Autodesk Fusion 360 part; units mm, degrees
(part 5 of 5)
sketch "Skizze81" plane through (0, 10, 0) normal (0, -1, 0) x (1, 0, 0)
  line L0 (-37.5877, 27.75) -> (-34.4123, 27.75)
  line L1 (-34.4123, 27.75) -> (-32.8246, 25)
  line L2 (-32.8246, 25) -> (-34.4123, 22.25)
  line L3 (-34.4123, 22.25) -> (-37.5877, 22.25)
  line L4 (-37.5877, 22.25) -> (-39.1754, 25)
  line L5 (-39.1754, 25) -> (-37.5877, 27.75)
  line L6 (-32.5, 27.5) -> (-33.8276, 28.3587)
  arc A0 (-33.8276, 28.3587) -> (-36.0513, 21.0003) centre (-36, 25) ccw
  arc A1 (-34.4939, 20.8944) -> (-36.0513, 21.0003) centre (-36.233, 6.8289) ccw
  line L7 (-34.4939, 20.8944) -> (-34.4939, 21.2944)
  arc A2 (-34.4939, 21.2944) -> (-32.6769, 27.2265) centre (-36, 25) ccw
  line L8 (-32.6769, 27.2265) -> (-32.5, 27.5)
  circle A3 centre (-36, 25) radius 4
  line L9 (-34.4123, -27.75) -> (-37.5877, -27.75)
  line L10 (-37.5877, -27.75) -> (-39.1754, -25)
  line L11 (-39.1754, -25) -> (-37.5877, -22.25)
  line L12 (-37.5877, -22.25) -> (-34.4123, -22.25)
  line L13 (-34.4123, -22.25) -> (-32.8246, -25)
  line L14 (-32.8246, -25) -> (-34.4123, -27.75)
  arc A4 (-36.0513, -21.0003) -> (-33.8276, -28.3587) centre (-36, -25) ccw
  line L15 (-33.8276, -28.3587) -> (-32.5, -27.5)
  line L16 (-32.5, -27.5) -> (-32.6769, -27.2265)
  arc A5 (-32.6769, -27.2265) -> (-34.4939, -21.2944) centre (-36, -25) ccw
  line L17 (-34.4939, -21.2944) -> (-34.4939, -20.8944)
  arc A6 (-36.0513, -21.0003) -> (-34.4939, -20.8944) centre (-36.233, -6.8289) ccw
  circle A7 centre (-36, 25) radius 1.9
  arc A8 (-33.8276, 28.3587) -> (-36.0513, 21.0003) centre (-36, 25) ccw
  line L18 (-33.8276, 28.3587) -> (-32.5, 27.5)
  line L19 (-32.5, 27.5) -> (32.5, 27.5)
  line L20 (32.5, 27.5) -> (32.5, 19)
  line L21 (32.5, 19) -> (31, 19)
  line L22 (31, 19) -> (31, 26)
  line L23 (31, 26) -> (-31, 26)
  line L24 (-31, 26) -> (-31, 20)
  arc A9 (-31, 20) -> (-36.0513, 21.0003) centre (-36.233, 6.8289) ccw
  circle A10 centre (-36, 25) radius 1.9
  line L25 (-45.682, 18.318) -> (-44.6213, 17.2574)
  line L26 (-44.6213, 17.2574) -> (-41.8787, 20)
  line L27 (-41.8787, 20) -> (-31, 20)
  line L28 (-31, 20) -> (-31, 26)
  line L29 (-31, 26) -> (31, 26)
  line L30 (31, 26) -> (31, 19.2)
  line L31 (31, 19.2) -> (32.5, 19.2)
  line L32 (32.5, 19.2) -> (32.5, 27.5)
  line L33 (32.5, 27.5) -> (-32.5, 27.5)
  line L34 (-32.5, 27.5) -> (-33.8276, 28.3587)
  arc A11 (-33.8276, 28.3587) -> (-39.5022, 26.9326) centre (-36, 25) ccw
  line L35 (-39.5022, 26.9326) -> (-42.5, 21.5)
  line L36 (-42.5, 21.5) -> (-45.682, 18.318)
  circle A12 centre (-36, 25) radius 1.9
  line L37 (-47.8033, 16.1967) -> (-45.682, 18.318)
  line L38 (-47.8033, 16.1967) -> (-46.7426, 15.136)
  line L39 (-44.6213, 17.2574) -> (-46.7426, 15.136)
  line L40 (-44.6213, 17.2574) -> (-45.682, 18.318)
  line L41 (-57.5, 6.5) -> (-47.8033, 16.1967)
  line L42 (-46.7426, 15.136) -> (-47.8033, 16.1967)
  line L43 (-47.8033, 16.1967) -> (-57.5, 6.5)
  line L44 (-57.5, 6.5) -> (-57.5, 4)
  line L45 (-57.5, 4) -> (-51.5218, 4)
  line L46 (-51.5218, 4) -> (-51.5218, 10.3569)
  line L47 (-51.5218, 10.3569) -> (-46.7426, 15.136)
  line L48 (-51.5218, 4) -> (-57.5, 4)
  line L49 (-57.5, -4) -> (-57.5, 4)
  line L50 (-57.5, -4) -> (-51.5218, -4)
  line L51 (-51.5218, 4) -> (-51.5218, -4)
  line L52 (-47.8033, -16.1967) -> (-46.7426, -15.136)
  line L53 (-46.7426, -15.136) -> (-51.5218, -10.3569)
  line L54 (-51.5218, -10.3569) -> (-51.5218, -4)
  line L55 (-51.5218, -4) -> (-57.5, -4)
  line L56 (-57.5, -4) -> (-57.5, -6.5)
  line L57 (-57.5, -6.5) -> (-47.8033, -16.1967)
  line L58 (-45.682, -18.318) -> (-47.8033, -16.1967)
  line L59 (-45.682, -18.318) -> (-44.6213, -17.2574)
  line L60 (-46.7426, -15.136) -> (-44.6213, -17.2574)
  line L61 (-46.7426, -15.136) -> (-47.8033, -16.1967)
  circle A13 centre (-36, -25) radius 1.9
  line L62 (-44.6213, -17.2574) -> (-45.682, -18.318)
  line L63 (-45.682, -18.318) -> (-42.5, -21.5)
  line L64 (-42.5, -21.5) -> (-39.5022, -26.9326)
  arc A14 (-39.5022, -26.9326) -> (-33.8276, -28.3587) centre (-36, -25) ccw
  line L65 (-33.8276, -28.3587) -> (-32.5, -27.5)
  line L66 (-32.5, -27.5) -> (-18.7617, -27.5)
  line L67 (-18.7617, -27.5) -> (-18.7617, -26)
  line L68 (-18.7617, -26) -> (-23, -26)
  line L69 (-23, -26) -> (-31, -26)
  line L70 (-31, -26) -> (-31, -20)
  line L71 (-31, -20) -> (-41.8787, -20)
  line L72 (-41.8787, -20) -> (-44.6213, -17.2574)
  circle A15 centre (-36, -25) radius 4
  arc A16 (-36.0513, 21.0003) -> (-41.8787, 20) centre (-36.2598, 4.7412) ccw
  arc A17 (-41.8787, -20) -> (-36.0513, -21.0003) centre (-36.2598, -4.7412) ccw
  constraint concentric A0 A3
  constraint concentric A4 A15
  constraint tangent A4 A15
  constraint tangent A0 A3
  constraint coincident A0.end A1.end
  constraint coincident L26.end L27.start
  constraint tangent A3 A16
  constraint coincident A4.start A6.start
  constraint coincident L71.end L72.start
  constraint tangent A15 A17
extrude "Extrusion94" add sketch "Skizze81" along normal blind 10 separate body contours L0 L1 L2 L3 L4 L5 | A0 A2 A3 A8 A11 | A0 A3 A8 L25 L26 L35 L36 L40 A16 | L25 L37 L38 L39 L40 L42 | L38 L41 L42 L43 L44 L45 L46 L47 L48 | L45 L48 L49 L50 L51 L55 | L50 L52 L53 L54 L55 L56 L57 L61 | L52 L58 L59 L60 L61 L62 | A4 L59 L62 L63 L64 L72 A15 A17 | A4 A5 A14 A15 | L9 L10 L11 L12 L13 L14 makes body 4
sketch "Skizze82" plane through (0, 10, 0) normal (0, 1, 0) x (-1, 0, 0)
  circle A0 centre (36, -25) radius 1.9
  circle A1 centre (36, 25) radius 1.9
  line L0 (51.5218, -10.3569) -> (41.8787, -20)
  arc A2 (36.0513, -21.0003) -> (41.8787, -20) centre (36.2598, -4.7412) ccw
  arc A3 (36.0513, -21.0003) -> (39.5022, -26.9326) centre (36, -25) ccw
  line L1 (39.5022, -26.9326) -> (42.5, -21.5)
  line L2 (42.5, -21.5) -> (57.5, -6.5)
  line L3 (57.5, -6.5) -> (57.5, 6.5)
  line L4 (57.5, 6.5) -> (42.5, 21.5)
  line L5 (42.5, 21.5) -> (39.5022, 26.9326)
  arc A4 (39.5022, 26.9326) -> (36.0513, 21.0003) centre (36, 25) ccw
  arc A5 (41.8787, 20) -> (36.0513, 21.0003) centre (36.2598, 4.7412) ccw
  line L6 (41.8787, 20) -> (51.5218, 10.3569)
  line L7 (51.5218, 10.3569) -> (51.5218, -10.3569)
  arc A6 (36.0513, 21.0003) -> (33.8276, 28.3587) centre (36, 25) ccw
  line L8 (33.8276, 28.3587) -> (32.5, 27.5)
  line L9 (32.5, 27.5) -> (-32.5, 27.5)
  line L10 (-32.5, 27.5) -> (-32.5, 19)
  line L11 (-32.5, 19) -> (-31, 19)
  line L12 (-31, 19) -> (-31, 26)
  line L13 (-31, 26) -> (31, 26)
  line L14 (31, 26) -> (31, 20)
  arc A7 (36.0513, 21.0003) -> (31, 20) centre (36.233, 6.8289) ccw
  circle A8 centre (36, 25) radius 1.9
  circle A9 centre (36, -25) radius 1.9
  circle A10 centre (36, 25) radius 1.9
  line L15 (41.8787, -20) -> (51.5218, -10.3569)
  line L16 (51.5218, -10.3569) -> (51.5218, 10.3569)
  line L17 (51.5218, 10.3569) -> (41.8787, 20)
  arc A11 (41.8787, 20) -> (36.0513, 21.0003) centre (36.2598, 4.7412) ccw
  arc A12 (39.5022, 26.9326) -> (36.0513, 21.0003) centre (36, 25) ccw
  line L18 (39.5022, 26.9326) -> (42.5, 21.5)
  line L19 (42.5, 21.5) -> (57.5, 6.5)
  line L20 (57.5, 6.5) -> (57.5, -6.5)
  line L21 (57.5, -6.5) -> (42.5, -21.5)
  line L22 (42.5, -21.5) -> (39.5022, -26.9326)
  arc A13 (36.0513, -21.0003) -> (39.5022, -26.9326) centre (36, -25) ccw
  arc A14 (36.0513, -21.0003) -> (41.8787, -20) centre (36.2598, -4.7412) ccw
  circle A15 centre (36, -25) radius 1.9
  arc A16 (33.8276, -28.3587) -> (36.0513, -21.0003) centre (36, -25) ccw
  arc A17 (31, -20) -> (36.0513, -21.0003) centre (36.233, -6.8289) ccw
  line L23 (31, -20) -> (31, -26)
  line L24 (31, -26) -> (18.7617, -26)
  line L25 (18.7617, -26) -> (18.7617, -27.5)
  line L26 (18.7617, -27.5) -> (32.5, -27.5)
  line L27 (32.5, -27.5) -> (33.8276, -28.3587)
  line L28 (39.9936, -25.2256) -> (40.3068, -25.4745)
  line L29 (37.6237, -21.3444) -> (37.6237, -20.9444)
  line L30 (0, 1.75) -> (0, 22.5)
  line L31 (-1.75, 0) -> (-22.5, 0)
  line L32 (39.9936, 25.2256) -> (40.3068, 25.4745)
  line L33 (37.6237, 21.3444) -> (37.6237, 20.9444)
  dimension "d393" = 0.4
  dimension "d394" = 0.4
  constraint coincident A16 L28.start
  constraint coincident L22 L28.end
  constraint coincident A16 L29.start
  constraint coincident A14 L29.end
  constraint parallel L29 L30
  constraint symmetric L28.start L31 L32.start
  constraint symmetric L28.end L31 L32.end
  constraint symmetric L29.start L31 L33.start
  constraint symmetric L29.end L31 L33.end
  measures "d393" distance of L28.start L28.end
  measures "d394" vertical distance of L29.start L29.end
extrude "Extrusion95" add sketch "Skizze82" along normal blind 9 contours L0 A2 L1 L2 L3 L4 L5 A5 L6 L7 A6 L15 L16 L17 A11 L18 L19 L20 L21 L22 A14 A16 L28 L29 L32 L33 bodies 4
sketch "Skizze83" plane through (0, 0, 0) normal (0, -1, 0) x (1, 0, 0)
  circle A0 centre (-36, -25) radius 1.9
  circle A1 centre (-36, 25) radius 1.9
  line L0 (-41.8787, -20) -> (-51.5218, -10.3569)
  line L1 (-51.5218, -10.3569) -> (-51.5218, 10.3569)
  line L2 (-51.5218, 10.3569) -> (-41.8787, 20)
  arc A2 (-36.0513, 21.0003) -> (-41.8787, 20) centre (-36.2598, 4.7412) ccw
  arc A3 (-36.0513, 21.0003) -> (-39.5022, 26.9326) centre (-36, 25) ccw
  line L3 (-39.5022, 26.9326) -> (-42.5, 21.5)
  line L4 (-42.5, 21.5) -> (-57.5, 6.5)
  line L5 (-57.5, 6.5) -> (-57.5, -6.5)
  line L6 (-57.5, -6.5) -> (-42.5, -21.5)
  line L7 (-42.5, -21.5) -> (-39.5022, -26.9326)
  arc A4 (-39.5022, -26.9326) -> (-36.0513, -21.0003) centre (-36, -25) ccw
  arc A5 (-41.8787, -20) -> (-36.0513, -21.0003) centre (-36.2598, -4.7412) ccw
  arc A6 (-31, -20) -> (-31, 20) centre (-45.151, 0) ccw
  arc A7 (-31, 20) -> (-34.4939, 20.8944) centre (-36.233, 6.8289) ccw
  arc A8 (-34.4939, -20.8944) -> (-31, -20) centre (-36.233, -6.8289) ccw
  arc A9 (-36.0513, -21.0003) -> (-34.4939, -20.8944) centre (-36.233, -6.8289) ccw
  arc A10 (-36.0513, 21.0003) -> (-39.5022, 26.9326) centre (-36, 25) ccw
  arc A11 (-34.4939, 20.8944) -> (-36.0513, 21.0003) centre (-36.233, 6.8289) ccw
  arc A12 (-39.9936, 25.2256) -> (-37.6237, 21.3444) centre (-36, 25) ccw
  line L8 (-37.6237, 21.3444) -> (-37.6237, 20.9444)
  arc A13 (-37.6237, 20.9444) -> (-41.8787, 20) centre (-36.2598, 4.7412) ccw
  line L9 (-41.8787, 20) -> (-51.5218, 10.3569)
  line L10 (-51.5218, 10.3569) -> (-51.5218, -10.3569)
  line L11 (-51.5218, -10.3569) -> (-41.8787, -20)
  arc A14 (-41.8787, -20) -> (-37.6237, -20.9444) centre (-36.2598, -4.7412) ccw
  line L12 (-37.6237, -20.9444) -> (-37.6237, -21.3444)
  arc A15 (-37.6237, -21.3444) -> (-39.9936, -25.2256) centre (-36, -25) ccw
  line L13 (-39.9936, -25.2256) -> (-40.3068, -25.4745)
  line L14 (-40.3068, -25.4745) -> (-42.5, -21.5)
  line L15 (-42.5, -21.5) -> (-57.5, -6.5)
  line L16 (-57.5, -6.5) -> (-57.5, 6.5)
  line L17 (-57.5, 6.5) -> (-42.5, 21.5)
  line L18 (-42.5, 21.5) -> (-40.3068, 25.4745)
  line L19 (-40.3068, 25.4745) -> (-39.9936, 25.2256)
extrude "Extrusion96" add sketch "Skizze83" against normal blind 3 contours L0 L1 L2 A2 A5 A6 A7 A8 A9 A11 A13 L9 L10 L11 A14 bodies 4
sketch "Skizze84" plane through (-57.5, 0, 0) normal (-1, 0, 0) x (0, 0, 1)
  line L0 (-6.5, 19) -> (-6.5, 0)
  line L1 (-6.5, 0) -> (6.5, 0)
  line L2 (6.5, 0) -> (6.5, 19)
  line L3 (6.5, 19) -> (-6.5, 19)
  arc A0 (4, 19) -> (-4, 19) centre (0, 19) ccw
  circle A1 centre (0, 19) radius 4
  constraint concentric A0 A1
  constraint tangent A0 A1
extrude "Extrusion97" cut sketch "Skizze84" against normal blind 6 contours L3 A1 bodies 4
sketch "Skizze85" plane through (0, 0, 0) normal (0, -1, 0) x (1, 0, 0)
  circle A0 centre (-36, -25) radius 1.9
  circle A1 centre (-36, 25) radius 1.9
  arc A2 (-36.0513, 21.0003) -> (-39.5022, 26.9326) centre (-36, 25) ccw
  line L0 (-39.5022, 26.9326) -> (-42.5, 21.5)
  line L1 (-42.5, 21.5) -> (-57.5, 6.5)
  line L2 (-57.5, 6.5) -> (-57.5, -6.5)
  line L3 (-57.5, -6.5) -> (-42.5, -21.5)
  line L4 (-42.5, -21.5) -> (-39.5022, -26.9326)
  arc A3 (-39.5022, -26.9326) -> (-36.0513, -21.0003) centre (-36, -25) ccw
  arc A4 (-36.0513, -21.0003) -> (-31, -20) centre (-36.233, -6.8289) ccw
  arc A5 (-31, -20) -> (-31, 20) centre (-45.151, 0) ccw
  arc A6 (-31, 20) -> (-36.0513, 21.0003) centre (-36.233, 6.8289) ccw
  line L5 (-34.4123, -27.75) -> (-32.8246, -25)
  line L6 (-32.8246, -25) -> (-34.4123, -22.25)
  line L7 (-34.4123, -22.25) -> (-37.5877, -22.25)
  line L8 (-37.5877, -22.25) -> (-39.1754, -25)
  line L9 (-39.1754, -25) -> (-37.5877, -27.75)
  line L10 (-37.5877, -27.75) -> (-34.4123, -27.75)
  line L11 (-37.5877, 22.25) -> (-34.4123, 22.25)
  line L12 (-34.4123, 22.25) -> (-32.8246, 25)
  line L13 (-32.8246, 25) -> (-34.4123, 27.75)
  line L14 (-34.4123, 27.75) -> (-37.5877, 27.75)
  line L15 (-37.5877, 27.75) -> (-39.1754, 25)
  line L16 (-39.1754, 25) -> (-37.5877, 22.25)
extrude "Extrusion98" cut sketch "Skizze85" against normal blind 3 contours L5 L6 L7 L8 L9 L10 | L11 L12 L13 L14 L15 L16 bodies 4
chamfer "Fase4" distance 0.85 angle 45 6 edges at (37.7714, 3, 15.1871) (37.7714, 3, -13.8129) (-34.2286, 13, 25.6871) (-34.2286, 13, -24.3129) (-37.7714, 3, 24.3129) (-37.7714, 3, -25.6871) on bodies 1 4
extrude "Extrusion99" add 6 faces at (16, 45, -39.6) (18.3333, 40.4869, -39.6) (18.3333, 3.6667, -39.6) (-18.3333, 3.6667, -39.6) (-19, 45, -39.6) (-18.3333, 40.4, -39.6) along direction (0, 0, -1) blind 1 on bodies 1 2 bodies 2 1 4
extrude "Extrusion100" cut 7 faces at (-20.0333, 37.3333, -38.1) (-15.4315, 42.1333, -38.1) (-17.7315, 39.6667, -38.1) (-17.7, 4.3333, -38.1) (17.7, 4.3333, -38.1) (17.7339, 39.7535, -38.1) (15.4006, 42.1333, -38.1) along direction (0, 0, -1) blind 1 on bodies 1 2 bodies 1 2
equation "d18 = d17"
equation "d19 = d17"
equation "d20 = d17"
equation "d24 = d23"
equation "d25 = d23"
equation "d26 = d23"
equation "d42 = d41"
equation "d43 = d41"
equation "d44 = d41"
equation "d45 = d41"
equation "d46 = d41"
equation "d47 = d41"
equation "d48 = d41"
equation "d49 = d41"
equation "d50 = d41"
equation "d51 = d41"
equation "d52 = d41"
equation "d53 = d41"
equation "d54 = d41"
equation "d98 = d95 / 2"
equation "d99 = d96 / 2"
equation "d198 = d197"
equation "d199 = d197"
equation "d200 = d197"
equation "d229 = d224 / 2"
equation "d230 = d225 / 2"
equation "d231 = ( d225 - 32 mm ) / 2"
equation "d232 = d231"
equation "d233 = d228"
equation "d234 = d231"
equation "d235 = d231"
named bodies: "Case_bottom", "Case_top", "Rotary_Knob", "Case_front"
